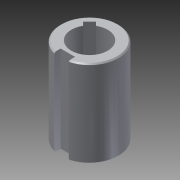
# Autodesk Inventor part: 0.5 inch Shaft to 8mm Shaft Insert
Saved by Autodesk Inventor 2014 SP1 (Build 180222100, 222)
## iProperties
Created: 2013-12-13
Part Number: 0.5 inch Shaft to 8mm Shaft Insert
Material: Aluminum 6061
Document SubType Name: Modeling
Designer: Moses
Density: 2.71 g/cm^3
Appearance: Aluminum - Flat
Mass: 3.5816 g
Surface Area: 14.613 cm^2
Volume: 1.32162 cm^3
Author: Moses
Autodesk Inventor part; units mm, degrees
ref_plane "YZ Plane" through (0, 0, 0) normal (1, 0, 0) x (0, 1, 0)
ref_plane "XZ Plane" through (0, 0, 0) normal (0, 1, 0) x (-1, 0, 0)
ref_plane "XY Plane" through (0, 0, 0) normal (0, 0, 1) x (1, 0, 0)
sketch "Sketch1" plane through (0, 0, 0) normal (0, 1, 0) x (-1, 0, 0)
  circle A0 centre (0, 0) radius 6.35
  circle A1 centre (0, 0) radius 4
  line L0 (-1.5875, 6.1484) -> (-1.5875, 4.7625)
  line L1 (-1.5875, 4.7625) -> (1.5875, 4.7625)
  line L2 (1.5875, 4.7625) -> (1.5875, 6.1484)
  line L3 (0, 6.35) -> (0, 0) construction
  line L4 (0, 0) -> (4.4901, -4.4901) construction
  line L5 (0, 0) -> (6.35, 0) construction
  line L6 (2.0315, -3.4457) -> (2.8284, -4.2426)
  line L7 (2.8284, -4.2426) -> (4.2426, -2.8284)
  line L8 (4.2426, -2.8284) -> (3.4457, -2.0315)
  line L9 (2.8284, -2.8284) -> (3.5355, -3.5355) construction
  point P0 (0, 4.7625)
  dimension "d0" = 12.7
  dimension "d1" = 8
  dimension "d4" = 3.175
  dimension "d5" = 45
  dimension "d6" = 2
  dimension "d8" = 1.5875
  dimension "d9" = 1
  constraints: 20 end point, 7 point on circle, 3 point on line, 3 vertical, 2 centre point, 2 coincident, 2 horizontal, 2 midpoint, 2 parallel, 1 collinear, 1 equal length, 1 perpendicular
  measures "d0" diameter of A0
  measures "d1" diameter of A1
  measures "d4" distance of L0.end L1.end
  measures "d5" angle of L4 L5
  measures "d6" distance of L6.end L7.end
  measures "d8" distance from line of L1 L3.start
  measures "d9" distance of L9.start L9.end
extrude "Extrusion1" add sketch "Sketch1" along normal blind 19.05 contours A0 L0 L1 L2 picked at (1.2402, -5.3906)
chamfer "Chamfer1" distance 0.254 angle 45 2 edges at (0, 19.05, -6.35) (0, 0, -6.35)
body "Solid1"
